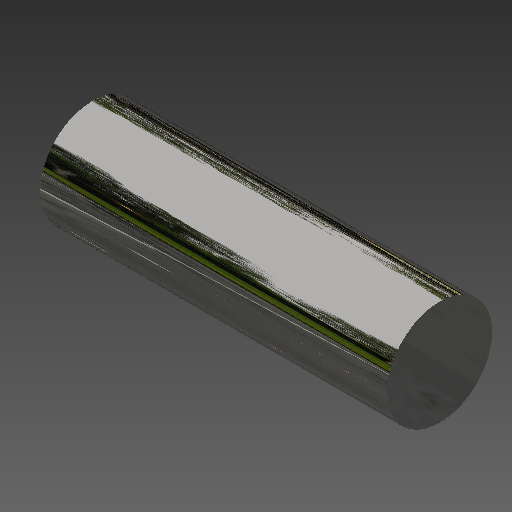
# Autodesk Inventor part: 3d_LM-Welding_Tooling -  4x14 Guide Pin
Saved by Autodesk Inventor 2018.3 (Build 223284000, 284)
## iProperties
Created: 2026-01-26
Part Number: 3d_LM-Welding_Tooling -  4x14 Guide Pin
Material: 304 Stainless Steel
Document SubType Name: Modeling
Designer: aca6
Density: 8 g/cm^3
Appearance: N/A - Machined Stainless Steel
Manufacturer-1: {"Name": "FABORY SPAIN S.L.U.\n", "PartNumber": "3d_Welding_Tooling -  4x14 Guide Pin", "Link": "https://www.fabory.com/es/pasador-din-7-m6-acero-inoxidable-%28inox%29-a1-a2-4x14mm-sku/p/51580040014"}
Manufacturer-2: {"Name": "", "PartNumber": "", "Link": ""}
Manufacturer-3: {"Name": "", "PartNumber": "", "Link": ""}
Manufacturer-4: {"Name": "", "PartNumber": "", "Link": ""}
Manufacturer-5: {"Name": "", "PartNumber": "", "Link": ""}
Provider-1: {"Name": "FABORY SPAIN S.L.U.", "PartNumber": "3d_Welding_Tooling -  4x14 Guide Pin", "Link": "https://www.fabory.com/es/pasador-din-7-m6-acero-inoxidable-%28inox%29-a1-a2-4x14mm-sku/p/51580040014"}
Provider-2: {"Name": "", "PartNumber": "", "Link": ""}
Provider-3: {"Name": "", "PartNumber": "", "Link": ""}
Provider-4: {"Name": "", "PartNumber": "", "Link": ""}
Provider-5: {"Name": "", "PartNumber": "", "Link": ""}
Author: aca6
Autodesk Inventor part; units mm, degrees
ref_plane "YZ Plane" through (0, 0, 0) normal (1, 0, 0) x (0, 1, 0)
ref_plane "XZ Plane" through (0, 0, 0) normal (0, 1, 0) x (-1, 0, 0)
ref_plane "XY Plane" through (0, 0, 0) normal (0, 0, 1) x (1, 0, 0)
sketch "Sketch1" plane through (0, 0, 0) normal (0, 0, 1) x (1, 0, 0)
  line L0 (-8.4076, 2) -> (4.8284, 2)
  line L1 (4.8284, 2) -> (4.8284, 0)
  line L2 (4.8284, 0) -> (-9.1716, 0)
  line L3 (-8.4076, 0) -> (-8.4076, 2)
  line L4 (0, 0) -> (3.6926, 0)
  line L5 (4.8284, 0) -> (9.1716, 0)
  arc A0 (-8.4076, 2) -> (-8.4076, -2) centre (-6.1716, 0) ccw
  line L6 (0, 0) -> (0, 0.5) construction
  dimension "d0" = 2
  dimension "d1" = 4
  dimension "d2" = 3
  dimension "d3" = 14
  constraints: 14 end point, 3 horizontal, 3 point on circle, 3 point on line, 3 vertical, 2 perpendicular, 1 centre point, 1 symmetric about line, 2 other
  measures "d0" distance of L0.end L1.end
  measures "d1" distance of L0.start A0.end
  measures "d2" radius of A0
  measures "d3" distance from line of L2.end L1
revolve "Revolution1" add sketch "Sketch1" angle 360 about axis through (0, 0, 0) along (1, 0, 0)
body "Solid1"
